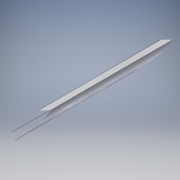
# Autodesk Inventor part: soprte baterias
Saved by Autodesk Inventor 2016 (Build 200138000, 138)
## iProperties
Created: 2017-03-10
Part Number: soprte baterias
Material: Generic
Document SubType Name: Modeling
Designer: jorge
Density: 1 g/cm^3
Appearance: White
Author: jorge
Autodesk Inventor part; units mm, degrees
ref_plane "YZ Plane" through (0, 0, 0) normal (1, 0, 0) x (0, 1, 0)
ref_plane "XZ Plane" through (0, 0, 0) normal (0, 1, 0) x (-1, 0, 0)
ref_plane "XY Plane" through (0, 0, 0) normal (0, 0, 1) x (1, 0, 0)
sketch "Sketch1" plane through (0, 0, 0) normal (0, 0, 1) x (1, 0, 0)
  arc A0 (1.5257, 2.5779) -> (-13.7171, -10.3703) centre (-6.0957, -3.8962) ccw projected
  line L0 (15.1214, -13.427) -> (1.5257, 2.5779) projected
  arc A1 (-0.1214, -26.3753) -> (15.1214, -13.427) centre (7.5, -19.9011) ccw projected
  line L1 (-13.7171, -10.3703) -> (-0.1214, -26.3753) projected
  arc A2 (3.8121, 4.5202) -> (-16.0035, -12.3126) centre (-6.0957, -3.8962) ccw
  line L2 (-16.0035, -12.3126) -> (-2.4078, -28.3175)
  arc A3 (-2.4078, -28.3175) -> (17.4078, -11.4848) centre (7.5, -19.9011) ccw
  line L3 (17.4078, -11.4848) -> (3.8121, 4.5202)
  line L4 (-0.1214, -26.3753) -> (-2.4078, -28.3175)
  line L5 (-13.7171, -10.3703) -> (-16.0035, -12.3126)
  line L6 (15.1214, -13.427) -> (17.4078, -11.4848)
  line L7 (1.5257, 2.5779) -> (3.8121, 4.5202)
  line L8 (13.9741, -27.5225) -> (15.9164, -29.8089)
  line L9 (17.4078, -21.2558) -> (20.4292, -21.2558)
  line L10 (10.61, -3.4823) -> (12.5522, -5.7687)
  line L11 (12.5522, -5.7687) -> (8.6677, -1.1959)
  line L12 (8.6677, -1.1959) -> (13.2406, 2.6886)
  line L13 (13.2406, 2.6886) -> (17.1251, -1.8842)
  line L14 (17.1251, -1.8842) -> (12.5522, -5.7687)
  line L15 (-9.2056, -20.315) -> (-11.1479, -18.0286)
  line L16 (-11.1479, -18.0286) -> (-7.2634, -22.6014)
  line L17 (-7.2634, -22.6014) -> (-11.8362, -26.4859)
  line L18 (-11.8362, -26.4859) -> (-15.7207, -21.9131)
  line L19 (-15.7207, -21.9131) -> (-11.1479, -18.0286)
  point P0 (0, 0)
  dimension "d0" = 3
  dimension "d3" = 3
  dimension "d4" = 6
  dimension "d5" = 6
  dimension "d6" = 6
  dimension "d7" = 3
  dimension "d8" = 6
  constraints: 36 end point, 10 point on line, 8 point on circle, 3 perpendicular, 2 centre point, 2 midpoint, 1 horizontal, 1 parallel, 3 other
  measures "d0" distance between parallel lines of L0 L3
  measures "d3" distance of L10.start L10.end
  measures "d4" distance of L10.end L11.end
  measures "d5" distance of L11.end L12.end
  measures "d6" distance of L12.end L13.end
  measures "d7" distance of L15.start L15.end
  measures "d8" distance of L16.end L17.end
ref_plane "Work Plane1" through (-37.5, -62.3962, 69) normal (0, 0, -1) x (0, 1, 0)
ref_plane "Work Plane2" through (-37.5, -62.3962, 72) normal (0, 0, 1) x (1, 0, 0)
extrude "Extrusion1" add sketch "Sketch1" along normal up to surface (72 mm away) contours L9 A3 L8 A1
sketch "Sketch2" plane through (0, 0, 0) normal (0, 0, -1) x (-1, 0, 0)
  line L0 (-13.9741, -27.5225) -> (-15.9164, -29.8089) projected
  arc A0 (-17.4078, -21.2558) -> (-13.9741, -27.5225) centre (-7.5, -19.9011) ccw projected
  line L1 (-20.4292, -21.2558) -> (-17.4078, -21.2558) projected
  arc A1 (-20.4292, -21.2558) -> (-15.9164, -29.8089) centre (-7.5, -19.9011) ccw projected
  point P0 (0, 0)
ref_plane "Work Plane3" through (-37.5, -15.3962, -3) normal (0, 0, -1) x (0, 1, 0)
extrude "Extrusion2" add sketch "Sketch2" along normal up to surface (3 mm away)
body "Solid1"
